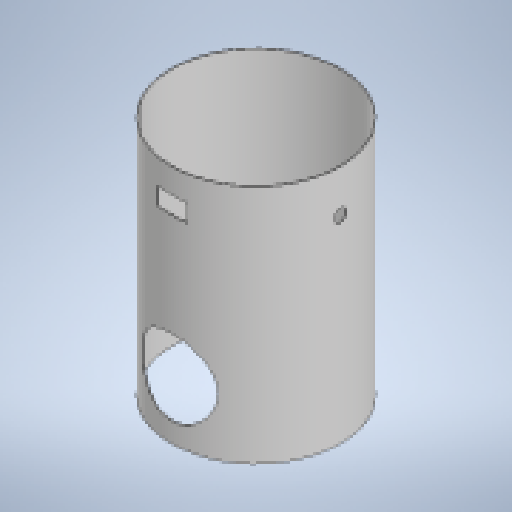
# Autodesk Inventor part: PRS 940-10 main Shell D 940
Saved by Autodesk Inventor 2025.4 (Build 294407000, 407)
## iProperties
Created: 2025-02-11
Part Number: PRS 940-10 main Shell D 940
Material: Steel
Document SubType Name: Sheet Metal
Designer: pokla
Mass: 197479 g
Surface Area: 84554.1 cm^2
Volume: 25156.5 cm^3
Density: 7.85 g/cm^3
Flat Pattern Width: 170 cm
Flat Pattern Length: 374.776 cm
Flat Pattern Area: 63711.9 cm^2
Sheet Metal Rule: Default_mm
Sheet Metal Width: 1700,000 mm
Sheet Metal Length: 3747,758 mm
Sheet Metal Area: 6371189,192 mm^2
Appearance: Default
Author: pokla
Autodesk Inventor part; units mm, degrees
sketch "Sketch13" plane through (0, 0, 0) normal (0, 0, 1) x (1, 0, 0)
  circle A0 centre (0, 0) radius 600 construction
  line L0 (0, 0) -> (0, -600)
  line L1 (0, 0) -> (-508.8289, -317.9516)
  line L2 (0, 0) -> (600, 0)
  line L3 (0, 0) -> (0, -600)
  line L4 (0, 0) -> (0, -600)
  line L5 (0, 0) -> (-534.6039, -272.3943)
  arc A1 (-508.8289, -317.9516) -> (0, -600) centre (0, 0) ccw
  dimension "d53" = 1200
  dimension "d54" = 58
  dimension "d55" = 0
  dimension "d56" = 0
  dimension "d57" = 270
  dimension "d58" = 63
  constraints: 12 end point, 8 point on circle, 2 centre point, 2 coincident, 1 vertical
  measures "d53" diameter of A0
  measures "d54" angle of L0 L1
  measures "d55" distance between parallel lines of L0 L4
  measures "d56" distance between parallel lines of L0 L3
  measures "d58" angle of L0 L5
ref_plane "WeldJoint" through (0, 0, -10) normal (0.5299, -0.848, 0) x (0, 0, 1)
ref_plane "Outer" through (0, 0, -10) normal (0.454, -0.891, 0) x (0, 0, 1)
ref_plane "Clock_Feeder" through (0, 0, -10) normal (0, 1, 0) x (0, 0, 1)
ref_plane "Charging" through (0, 0, -10) normal (1, 0, 0) x (0, 0, 1)
ref_plane "Accsess" through (0, 0, -10) normal (1, 0, 0) x (0, 0, 1)
sketch "Sketch14" plane through (0, 0, -10) normal (0.5299, -0.848, 0) x (0, 0, 1)
  line L0 (1710, 594) -> (10, 594)
  line L1 (10, 594) -> (10, 600)
  line L2 (10, 600) -> (1710, 600)
  line L3 (1710, 600) -> (1710, 594)
  line L4 (10, 0) -> (825.0673, 0)
  point P0 (10, 597)
  dimension "d59" = 1700
  dimension "d60" = 6
  dimension "d61" = 1200
  constraints: 10 end point, 2 horizontal, 2 parallel, 1 midpoint, 1 perpendicular, 1 vertical alignment
  measures "d59" distance of L1.end L2.end
  measures "d60" distance of L0.end L1.end
  measures "d61" diameter of L2 L4
revolve "Revolution2" add sketch "Sketch14" angle 359.9 about axis through (0, 0, 0) along (0, 0, 1)
sketch "Sketch AnglePlane_Feeder" plane through (0, 0, -10) normal (0, 1, 0) x (0, 0, 1)
  line L0 (10, -600) -> (10, 600) projected
  line L1 (10, 0) -> (1410, 0)
  line L2 (1410, 0) -> (1410, 600)
  line L3 (1410, 600) -> (10, 600)
  line L4 (10, 600) -> (10, 0)
  point P0 (10, -508.8289)
  point P1 (10, -509.383)
  dimension "d63" = 1200
  dimension "d64" = 90
  dimension "frd_hght" = 1400
  constraints: 8 end point, 1 collinear, 1 horizontal, 1 parallel
  measures "d63" diameter of L3 L1
  measures "d64" angle of L2 L3
  measures "frd_hght" distance of L2.end L3.end
ref_plane "AnglePlane_Feeder" through (0, 0, 1400) normal (1, 0, 0) x (0, 1, 0)
sketch "Sketch16" plane through (0, 0, 1400) normal (1, 0, 0) x (0, 1, 0)
  circle A0 centre (0, 0) radius 45.5
  point P0 (0, -1400)
  point P1 (0, 0)
  point P2 (0, 0)
  point P3 (0, 0)
  dimension "d66" = 91
  constraints: 1 centre point, 1 coincident
  measures "d66" diameter of A0
extrude "Extrusion7" cut sketch "Sketch16" along normal through all
ref_plane "Work Plane16" through (0, 0, 0) normal (0, -1, 0) x (1, 0, 0)
sketch "Sketch17" plane through (0, 0, 0) normal (0, -1, 0) x (1, 0, 0)
  circle A0 centre (0, 408.5) radius 268.5
  line L0 (0, 140) -> (-495.5727, 140)
  point P0 (0, 0)
  dimension "d69" = 537
  dimension "d71" = 140
  constraints: 2 end point, 2 horizontal, 2 vertical alignment, 2 other
  measures "d71" distance from line of point (0, 0) L0
extrude "Extrusion8" cut sketch "Sketch17" along normal through all
sketch "Sketch19" plane through (0, 0, -10) normal (1, 0, 0) x (0, 0, 1)
  line L0 (10, 0) -> (1410, 0)
  line L1 (1410, 0) -> (1410, 600)
  line L2 (1410, 600) -> (10, 600)
  line L3 (10, 600) -> (10, 0)
  dimension "d74" = 1400
  dimension "d76" = 1200
  dimension "d77" = 90
  constraints: 8 end point, 1 horizontal, 1 parallel, 1 perpendicular
  measures "d74" distance of L1.end L2.end
  measures "d76" diameter of L2 L0
  measures "d77" angle of L2 L1
ref_plane "Work Plane18" through (0, 0, 1400) normal (0, -1, 0) x (1, 0, 0)
sketch "Sketch20" plane through (0, 0, 1400) normal (0, -1, 0) x (1, 0, 0)
  line L0 (-103.5, 0) -> (103.5, 0)
  line L1 (103.5, 0) -> (103.5, 125)
  line L2 (103.5, 125) -> (-103.5, 125)
  line L3 (-103.5, 125) -> (-103.5, 0)
  point P0 (0, -1400)
  point P1 (0, 0)
  point P2 (0, 0)
  point P3 (0, 0)
  point P4 (0, 0)
  dimension "d78" = 207
  dimension "d79" = 125
  constraints: 8 end point, 2 parallel, 1 coincident, 1 horizontal, 1 midpoint, 1 perpendicular
  measures "d78" distance of L2.end L1.end
  measures "d79" distance of L1.end L0.end
extrude "Extrusion9" cut sketch "Sketch20" along normal through all
equation "\"BendRadius\" = Thickness"
equation "\"BendReliefWidth\" = Thickness"
equation "\"BendReliefDepth\" = 0.5 * Thickness"
equation "\"CornerReliefSize\" = 4 * Thickness"
equation "\"MinimumRemnant\" = 2 * Thickness"
equation "\"TransitionRadius\" = BendRadius"
equation "\"JacobiRadiusSize\" = BendRadius"
equation "\"GapSize\" = Thickness"
equation "\"Feeder_horisont_angle\" = 0"
equation "\"Hatch_Accsess_diameter\" = 535"
equation "\"Clock_Accsess_angle\" = 0"
equation "\"Clock_Charging_agnle\" = 0"
equation "\"Clock_Feeder_angle\" = 270deg"
equation "\"Clock_Outer_angle\" = 63deg"
equation "\"Clock_WeldJoint_angle\" = 58deg"
equation "\"Thickness\" = 6"
body "Solid2"
